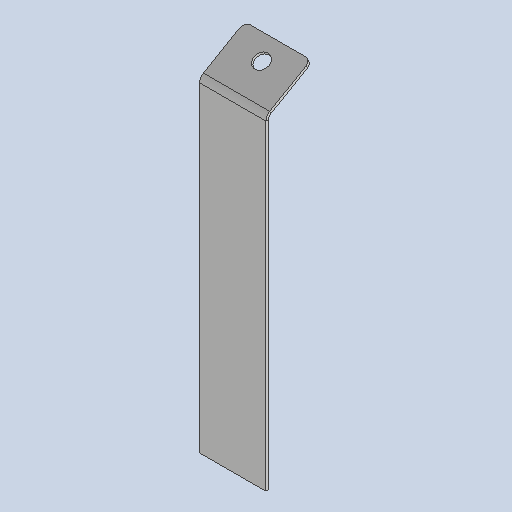
# Autodesk Inventor part: MSC 202 GRID CORNER
Saved by Autodesk Inventor 2025 (Build 290162010, 162A)
## iProperties
Created: 2025-01-14
Part Number: MSC 202 GRID CORNER
Material: Stainless Steel
Document SubType Name: Sheet Metal
Designer: pokla
Density: 8 g/cm^3
Sheet Metal Rule: AISI304 3mm Die 32
Appearance: Default
Mass: 659.36 g
Surface Area: 578.754 cm^2
Volume: 82.42 cm^3
Flat Pattern Width: 7 cm
Flat Pattern Length: 39.5381 cm
Flat Pattern Area: 276.766 cm^2
Sheet Metal Width: 70,000 mm
Sheet Metal Length: 395,381 mm
Sheet Metal Area: 27676,648 mm^2
Author: pokla
Autodesk Inventor part; units mm, degrees
ref_plane "YZ Plane" through (0, 0, 0) normal (1, 0, 0) x (0, 1, 0)
ref_plane "XZ Plane" through (0, 0, 0) normal (0, 1, 0) x (-1, 0, 0)
ref_plane "XY Plane" through (0, 0, 0) normal (0, 0, 1) x (1, 0, 0)
sketch "Sketch1" plane through (0, 0, 0) normal (0, 1, 0) x (-1, 0, 0)
  line L0 (35, 0) -> (-35, 0)
  line L1 (-35, 0) -> (-35, 343)
  line L2 (-35, 343) -> (35, 343)
  line L3 (35, 343) -> (35, 0)
  point P0 (0, 0)
  point P1 (0, 0)
  point P2 (0, 0)
  dimension "d7" = 70
  dimension "d8" = 343
  measures "d7" distance of L0.start L0.end
  measures "d8" distance of L0.end L1.end
extrude "Plate1" add sketch "Sketch1" along normal mid plane 3
sketch "Sketch2" plane through (35, 0, 340.4019) normal (0, -0.5, 0.8660254) x (1, 0, 0)
  line L0 (-70, 0) -> (0, 0)
  line L1 (0, 0) -> (0, 55)
  line L2 (0, 55) -> (-70, 55)
  line L3 (-70, 55) -> (-70, 0)
  constraints: 6 end point, 1 horizontal, 1 perpendicular, 1 vertical
edge flange "Flange1" height 55 angle 60 thickness 3 bend radius 5 thickness toward (0, -0.5, 0.8660254) relief round relief width 3 relief depth 1.5 edges at (0, 1.5, 343) wall of the first edge with corners at (-35, 0, 340.4019) (35, 0, 340.4019) (35, 47.6314, 367.9019) (-35, 47.6314, 367.9019)
bend "Bend1"
corner "Corner1"
sketch "Sketch3" plane through (-35, 46.1314, 370.5) normal (0, -0.5, 0.8660254) x (1, 0, 0)
  circle A0 centre (35, -20) radius 8
  line L0 (0, 0) -> (70, 0) projected
  point P0 (35, -225.201)
  point P1 (35, 0)
  dimension "d19" = 20
  dimension "d20" = 16
  constraints: 1 centre point, 1 midpoint, 1 vertical alignment
  measures "d19" distance from line of L0 A0.centre
  measures "d20" diameter of A0
extrude "Cut1" cut sketch "Sketch3" against normal blind 3
fillet "Corner Round1" radius 6 2 edges at (35, 46.8814, 369.201) (-35, 46.8814, 369.201)
equation "\"d21\" = Thickness"
equation "\"d6\" = Thickness"
equation "\"d9\" = BendReliefWidth"
equation "\"d10\" = BendReliefDepth"
equation "\"d11\" = MinimumRemnant"
equation "\"d12\" = TransitionRadius"
equation "\"d15\" = BendRadius"
equation "\"d16\" = CornerReliefSize"
equation "\"d17\" = GapSize"
equation "\"d18\" = JacobiRadiusSize"
equation "\"BendReliefWidth\" = Thickness"
equation "\"BendReliefDepth\" = 0.5 * Thickness"
equation "\"CornerReliefSize\" = 4 * Thickness"
equation "\"MinimumRemnant\" = 2 * Thickness"
equation "\"TransitionRadius\" = BendRadius"
equation "\"JacobiRadiusSize\" = BendRadius"
equation "\"GapSize\" = Thickness"
equation "\"Thickness\" = 3"
equation "\"BendRadius\" = 5"
body "Solid1"
